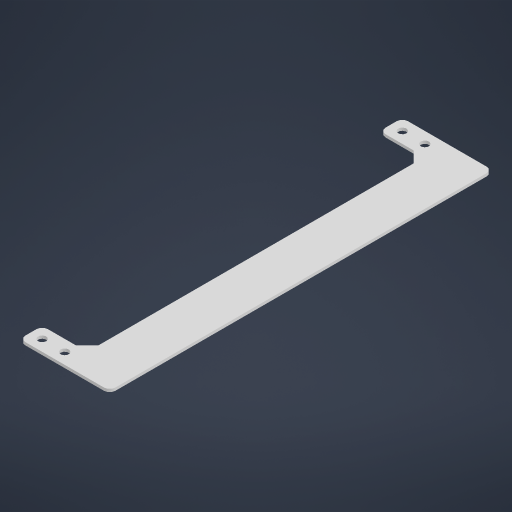
# Autodesk Inventor part: underside
Saved by Autodesk Inventor 2024 (Build 280153000, 153)
## iProperties
Created: 2023-12-14
Part Number: underside
Material: Generic
Document SubType Name: Sheet Metal
Designer: reima
Density: 1 g/cm^3
Sheet Metal Rule: Default
Appearance: Default
Author: reima
Autodesk Inventor part; units mm, degrees
ref_plane "YZ Plane" through (0, 0, 0) normal (1, 0, 0) x (0, 1, 0)
ref_plane "XZ Plane" through (0, 0, 0) normal (0, 1, 0) x (-1, 0, 0)
ref_plane "XY Plane" through (0, 0, 0) normal (0, 0, 1) x (1, 0, 0)
sketch "Sketch1" plane through (0, 0, 0) normal (0, 1, 0) x (-1, 0, 0)
  line L0 (-5.9237, 13.0609) -> (-28.1487, 13.0609)
  line L1 (-31.3237, 9.8859) -> (-31.3237, -199.6641)
  line L2 (-28.1487, -202.8391) -> (-5.9237, -202.8391)
  line L3 (-5.9237, -186.9641) -> (-5.9237, -2.8141)
  line L4 (-5.9237, 13.0609) -> (3.6013, 13.0609)
  line L5 (6.7763, 9.8859) -> (6.7763, 3.5359)
  line L6 (3.6013, 0.3609) -> (-2.7487, 0.3609)
  line L7 (-5.9237, 0.3609) -> (-5.9237, 13.0609)
  line L8 (-5.9237, -202.8391) -> (3.6013, -202.8391)
  line L9 (6.7763, -199.6641) -> (6.7763, -193.3141)
  line L10 (3.6013, -190.1391) -> (-2.7487, -190.1391)
  line L11 (-5.9237, -190.1391) -> (-5.9237, -202.8391)
  arc A0 (3.6013, 0.3609) -> (6.7763, 3.5359) centre (3.6013, 3.5359) ccw
  arc A1 (-2.7487, 0.3609) -> (-5.9237, -2.8141) centre (-2.7487, -2.8141) ccw
  arc A2 (-5.9237, -186.9641) -> (-2.7487, -190.1391) centre (-2.7487, -186.9641) ccw
  arc A3 (6.7763, -193.3141) -> (3.6013, -190.1391) centre (3.6013, -193.3141) ccw
  arc A4 (3.6013, -202.8391) -> (6.7763, -199.6641) centre (3.6013, -199.6641) ccw
  arc A5 (-31.3237, -199.6641) -> (-28.1487, -202.8391) centre (-28.1487, -199.6641) ccw
  arc A6 (-28.1487, 13.0609) -> (-31.3237, 9.8859) centre (-28.1487, 9.8859) ccw
  arc A7 (6.7763, 9.8859) -> (3.6013, 13.0609) centre (3.6013, 9.8859) ccw
  circle A8 centre (0.4263, 6.7109) radius 2.3368
  circle A9 centre (0.4263, -196.4891) radius 2.3368
  circle A10 centre (-12.2737, 6.7109) radius 2.3368
  circle A11 centre (-12.2737, -196.4891) radius 2.3368
  point P0 (0, 0)
  point P1 (-31.3237, -202.8391)
  point P2 (-31.3237, 13.0609)
  point P3 (6.7763, 0.3609)
  point P4 (6.7763, 13.0609)
  point P5 (6.7763, -190.1391)
  point P6 (6.7763, -202.8391)
  point P7 (-17.0362, -202.8391)
  point P8 (6.7763, -196.4891)
  dimension "d0" = 25.4
  dimension "d1" = 215.9
  dimension "d2" = 12.7
  dimension "d3" = 12.7
  dimension "d4" = 12.7
  dimension "d5" = 12.7
  dimension "d6" = 3.175
  dimension "d7" = 4.6736
  dimension "d8" = 4.6736
  dimension "d9" = 6.35
  dimension "d10" = 6.35
  dimension "d11" = 203.2
  dimension "d12" = 6.35
  dimension "d13" = 4.6736
  dimension "d14" = 12.7
  dimension "d15" = 4.6736
  dimension "d16" = 12.7
  dimension "d17" = 203.2
  measures "d0" distance of L2.end point (-31.324, -202.839)
  measures "d1" distance of point (-31.324, -202.839) point (-31.324, 13.061)
  measures "d2" distance of point (6.776, 0.361) L7.start
  measures "d3" distance of point (6.776, 13.061) point (6.776, 0.361)
  measures "d4" distance of L11.start point (6.776, -190.139)
  measures "d5" distance of point (6.776, -190.139) point (6.776, -202.839)
  measures "d6" radius of A0
  measures "d7" diameter of A8
  measures "d8" diameter of A9
  measures "d9" vertical distance of point (-17.036, -202.839) A9.centre
  measures "d10" distance of point (6.776, -196.489) A9.centre
  measures "d11" distance of A9.centre A8.centre
  measures "d12" distance from line of L5 A8.centre
  measures "d13" diameter of A10
  measures "d14" distance of A8.centre A10.centre
  measures "d15" diameter of A11
  measures "d16" distance of A9.centre A11.centre
  measures "d17" distance of A10.centre A11.centre
sketch "Sketch2" plane through (0, 1.5875, 0) normal (0, 1, 0) x (1, 0, 0)
  line L0 (-3.6013, 202.8391) -> (-16.3013, 202.8391)
  line L1 (-19.4763, 199.6641) -> (-19.4763, 193.3141)
  line L2 (-16.3013, 190.1391) -> (-3.6013, 190.1391)
  line L3 (-3.6013, 190.1391) -> (-3.6013, 202.8391)
  line L4 (31.3237, 199.6641) -> (31.3237, -9.8859)
  arc A0 (-16.3013, 202.8391) -> (-19.4763, 199.6641) centre (-16.3013, 199.6641) ccw
  arc A1 (-19.4763, 193.3141) -> (-16.3013, 190.1391) centre (-16.3013, 193.3141) ccw
  circle A2 centre (-13.1263, 196.4891) radius 2.3368
  circle A3 centre (-0.4263, 196.4891) radius 2.3368
  circle A4 centre (12.2737, 196.4891) radius 2.3368
  circle A5 centre (12.2737, -6.7109) radius 2.3368
  circle A6 centre (-0.4263, -6.7109) radius 2.3368
  line L5 (-3.6013, -13.0609) -> (-16.3013, -13.0609)
  line L6 (-19.4763, -9.8859) -> (-19.4763, -3.5359)
  line L7 (-16.3013, -0.3609) -> (-3.6013, -0.3609)
  line L8 (-3.6013, -0.3609) -> (-3.6013, -13.0609)
  line L9 (-3.6013, -0.3609) -> (2.7487, -0.3609)
  circle A7 centre (-13.1263, -6.7109) radius 2.3368
  arc A8 (-16.3013, -0.3609) -> (-19.4763, -3.5359) centre (-16.3013, -3.5359) ccw
  arc A9 (-19.4763, -9.8859) -> (-16.3013, -13.0609) centre (-16.3013, -9.8859) ccw
  point P0 (0, 0)
  point P1 (-9.9513, -13.0609)
  dimension "d19" = 50.8
  dimension "d20" = 3.175
  dimension "d21" = 4.6736
  dimension "d22" = 12.7
  dimension "d23" = 6.35
  dimension "d24" = 0
  dimension "d25" = 4.6736
  dimension "d26" = 12.7
  dimension "d27" = 6.35
  dimension "d28" = 3.175
  measures "d19" distance between parallel lines of L4 L1
  measures "d20" radius of A0
  measures "d21" diameter of A2
  measures "d22" distance of A2.centre A3.centre
  measures "d23" distance from line of L2 A2.centre
  measures "d24" distance between parallel lines of L9 L7
  measures "d25" diameter of A7
  measures "d26" distance of A7.centre A6.centre
  measures "d27" vertical distance of point (-9.951, -13.061) A7.centre
  measures "d28" radius of A8
sketch "Sketch3" plane through (0, 1.5875, 0) normal (0, 1, 0) x (1, 0, 0)
  circle A0 centre (-0.4263, -6.7109) radius 2.3368
  circle A1 centre (-0.4263, 196.4891) radius 2.3368
  line L0 (-16.3013, 190.1391) -> (2.7487, 190.1391)
  line L1 (-0.4263, 190.1391) -> (5.9237, 183.7891)
  line L2 (5.9237, 2.8141) -> (5.9237, 186.9641)
  line L3 (-0.4263, 190.1391) -> (8.5539, 190.1391) construction
  line L4 (-16.3013, -0.3609) -> (2.7487, -0.3609)
  line L5 (-0.4263, -0.3609) -> (5.9237, 5.9891)
  line L6 (-0.4263, -0.3609) -> (8.5539, -0.3609) construction
  circle A2 centre (-13.1263, 196.4891) radius 2.3368
  circle A3 centre (-13.1263, -6.7109) radius 2.3368
  line L7 (-16.3013, 190.1391) -> (2.7487, 190.1391)
  arc A4 (5.9237, 186.9641) -> (2.7487, 190.1391) centre (2.7487, 186.9641) ccw
  line L8 (5.9237, 2.8141) -> (5.9237, 186.9641)
  arc A5 (2.7487, -0.3609) -> (5.9237, 2.8141) centre (2.7487, 2.8141) ccw
  line L9 (-16.3013, -0.3609) -> (2.7487, -0.3609)
  arc A6 (-16.3013, -0.3609) -> (-19.4763, -3.5359) centre (-16.3013, -3.5359) ccw
  line L10 (-19.4763, -3.5359) -> (-19.4763, -9.8859)
  arc A7 (-19.4763, -9.8859) -> (-16.3013, -13.0609) centre (-16.3013, -9.8859) ccw
  line L11 (-16.3013, -13.0609) -> (28.1487, -13.0609)
  arc A8 (28.1487, -13.0609) -> (31.3237, -9.8859) centre (28.1487, -9.8859) ccw
  line L12 (31.3237, 199.6641) -> (31.3237, -9.8859)
  arc A9 (31.3237, 199.6641) -> (28.1487, 202.8391) centre (28.1487, 199.6641) ccw
  line L13 (-16.3013, 202.8391) -> (28.1487, 202.8391)
  arc A10 (-16.3013, 202.8391) -> (-19.4763, 199.6641) centre (-16.3013, 199.6641) ccw
  line L14 (-19.4763, 199.6641) -> (-19.4763, 193.3141)
  arc A11 (-19.4763, 193.3141) -> (-16.3013, 190.1391) centre (-16.3013, 193.3141) ccw
  circle A12 centre (-0.4263, -6.7109) radius 2.3368
  circle A13 centre (-0.4263, 196.4891) radius 2.3368
  point P0 (0, 0)
  point P1 (2.7487, -0.3609)
  point P2 (2.7487, 190.1391)
  dimension "d34" = 45
  dimension "d35" = 45
  measures "d34" angle of L1 L3
  measures "d35" angle of L6 L5
extrude "Plate1" add sketch "Sketch1" along normal blind 1.5875
sheet face with bend "Face2" sketch "Sketch2" thickness 1.5875 toward (0, -1, 0) bend radius 1.5875 relief straight relief width 1.5875 relief depth 0.7937 contours L3 L2 A1 L1 A0 L0 | A4 | A5 | L5 A9 L6 A8 L7 L8
bend "Bend1"
sheet face with bend "Face3" sketch "Sketch3" thickness 1.5875 toward (0, -1, 0) bend radius 1.5875 relief straight relief width 1.5875 relief depth 0.7937 contours L0 A4 L2 L1 | L2 A5 L4 L5
bend "Bend2"
equation "\"d18\" = Thickness"
equation "\"d29\" = BendRadius"
equation "\"d30\" = BendReliefWidth"
equation "\"d32\" = MinimumRemnant"
equation "\"d31\" = BendReliefDepth"
equation "\"d33\" = TransitionRadius"
equation "\"d36\" = BendRadius"
equation "\"d37\" = BendReliefWidth"
equation "\"d39\" = MinimumRemnant"
equation "\"d38\" = BendReliefDepth"
equation "\"d40\" = TransitionRadius"
equation "\"BendRadius\" = Thickness"
equation "\"BendReliefWidth\" = Thickness"
equation "\"BendReliefDepth\" = 0.5 * Thickness"
equation "\"CornerReliefSize\" = 4 * Thickness"
equation "\"MinimumRemnant\" = 2 * Thickness"
equation "\"TransitionRadius\" = BendRadius"
equation "\"JacobiRadiusSize\" = BendRadius"
equation "\"GapSize\" = Thickness"
equation "\"Thickness\" = 1.5875"
body "Solid1"
